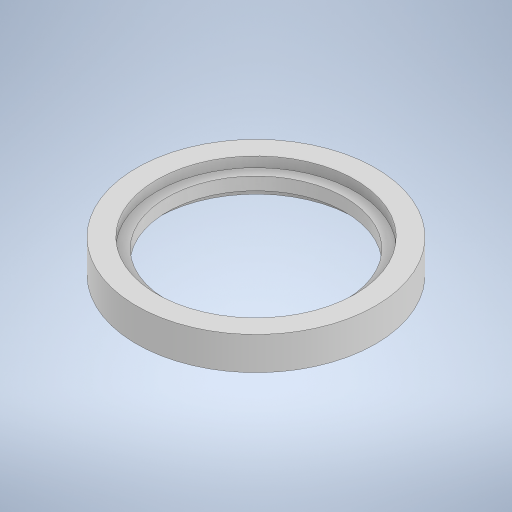
# Autodesk Inventor part: 3_AnilloPorSoldar
Saved by Autodesk Inventor 2024.3 (Build 283343000, 343)
## iProperties
Created: 2024-04-24
Part Number: 3_AnilloPorSoldar
Material: Genérico
Document SubType Name: Modeling
Designer: Cosmic Dinodog
Density: 1 g/cm^3
Appearance: Valor por defecto
Author: Cosmic Dinodog
Autodesk Inventor part; units mm, degrees
ref_plane "YZ Plane" through (0, 0, 0) normal (1, 0, 0) x (0, 1, 0)
ref_plane "XZ Plane" through (0, 0, 0) normal (0, 1, 0) x (-1, 0, 0)
ref_plane "XY Plane" through (0, 0, 0) normal (0, 0, 1) x (1, 0, 0)
sketch "Boceto1" plane through (0, 0, 0) normal (0, 0, 1) x (1, 0, 0)
  line L0 (0, 0) -> (47, 0) construction
  line L1 (47, 0) -> (47, 13)
  line L2 (47, 13) -> (39, 13)
  line L3 (39, 13) -> (39, 9)
  line L4 (39, 9) -> (35, 9)
  line L5 (35, 9) -> (35, 4)
  line L6 (35, 4) -> (39, 4)
  line L7 (39, 4) -> (39, 0)
  line L8 (39, 0) -> (47, 0)
  line L9 (0, 0) -> (0, 20.7267) construction
  dimension "d0" = 47
  dimension "d1" = 13
  dimension "d2" = 8
  dimension "d3" = 4
  dimension "d4" = 4
  dimension "d5" = 5
  dimension "d6" = 4
  constraints: 20 end point, 3 perpendicular, 3 point on line, 2 vertical, 1 collinear, 1 horizontal, 1 parallel
  measures "d0" distance of L0.start L0.end
  measures "d1" distance of L0.end L1.end
  measures "d2" distance of L1.end L2.end
  measures "d3" distance of L2.end L3.end
  measures "d4" distance of L3.end L4.end
  measures "d5" distance of L4.end L5.end
  measures "d6" distance of L5.end L6.end
revolve "Revolución1" add sketch "Boceto1" angle 360 about axis through (0, 0, 0) along (0, 1, 0)
